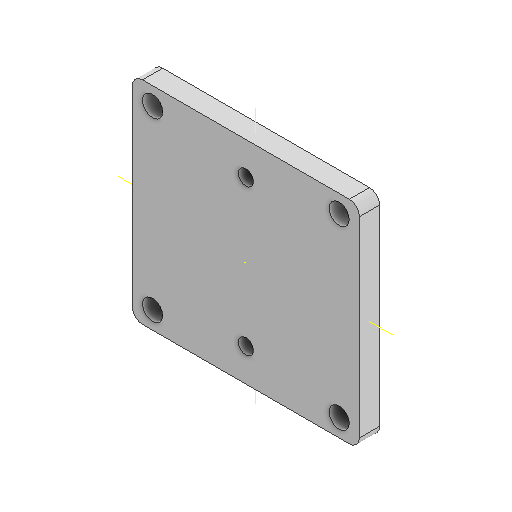
# Autodesk Inventor part: 집게_고정대
Saved by Autodesk Inventor 2027 (Build 310192000, 192)
## iProperties
Created: 2026-09-23
Part Number: 집게_고정대
Material: 일반
Document SubType Name: Modeling
Designer: User
Density: 1 g/cm^3
Appearance: 기본값
Author: User
Autodesk Inventor part; units mm, degrees
ref_plane "YZ 평면_우측면도" through (0, 0, 0) normal (1, 0, 0) x (0, 1, 0)
ref_plane "XZ 평면_평면도" through (0, 0, 0) normal (0, 1, 0) x (-1, 0, 0)
ref_plane "XY 평면_정면도" through (0, 0, 0) normal (0, 0, 1) x (1, 0, 0)
sketch "스케치1" plane through (0, 0, 0) normal (0, 0, 1) x (1, 0, 0)
  line L0 (20.5, -21) -> (-20.5, -21)
  line L1 (-22.5, -19) -> (-22.5, 19)
  line L2 (-20.5, 21) -> (20.5, 21)
  line L3 (22.5, 19) -> (22.5, -19)
  line L4 (22.5, -21) -> (-22.5, 21) construction
  line L5 (-22.5, -21) -> (22.5, 21) construction
  line L6 (0, 21) -> (0, -21) construction
  line L7 (-22.5, 14.5) -> (22.5, 14.5) construction
  circle A0 centre (0, 14.5) radius 1.5
  line L8 (-22.5, -14.5) -> (22.5, -14.5) construction
  circle A1 centre (0, -14.5) radius 1.5
  line L9 (-23.5, -17.5) -> (26.5, -17.5) construction
  line L10 (-23.5, 17.5) -> (26.5, 17.5) construction
  line L11 (-18.5, 21) -> (-18.5, -21) construction
  line L12 (18.5, 21) -> (18.5, -21) construction
  circle A2 centre (-18.5, 17.5) radius 2
  circle A3 centre (-18.5, -17.5) radius 2
  circle A4 centre (18.5, 17.5) radius 2
  circle A5 centre (18.5, -17.5) radius 2
  line L13 (-33.5, 0) -> (36.5, 0) projected
  line L14 (0, -29.9799) -> (0, 29.9799) projected
  arc A6 (-20.5, 21) -> (-22.5, 19) centre (-20.5, 19) ccw
  arc A7 (-22.5, -19) -> (-20.5, -21) centre (-20.5, -19) ccw
  arc A8 (20.5, -21) -> (22.5, -19) centre (20.5, -19) ccw
  arc A9 (22.5, 19) -> (20.5, 21) centre (20.5, 19) ccw
  point P0 (0, 0)
  dimension "d26" = 3
  dimension "d27" = 4
  dimension "d28" = 4
  dimension "d29" = 4
  dimension "d30" = 3
  dimension "d31" = 4
  dimension "d32" = 29
  dimension "d33" = 18.5
  dimension "d34" = 35
  dimension "d35" = 42
  dimension "d36" = 45
  dimension "d37" = 2
  constraints: 32 point on line, 26 end point, 10 centre point, 8 point on circle, 8 tangent, 6 midpoint, 4 parallel, 3 equal radius, 3 perpendicular, 2 horizontal, 1 collinear, 3 other
  measures "d26" diameter of A0
  measures "d27" diameter of A2
  measures "d28" diameter of A4
  measures "d29" diameter of A3
  measures "d30" diameter of A1
  measures "d31" diameter of A5
  measures "d32" distance between parallel lines of L8 L7
  measures "d33" distance between parallel lines of L6 L11
  measures "d34" distance between parallel lines of L9 L10
  measures "d35" distance between parallel lines of L0 L2
  measures "d36" distance between parallel lines of L3 L1
  measures "d37" radius of A6
extrude "돌출1" add sketch "스케치1" along normal mid plane 4 contours L0 L14 A1 L13 L3 A8 | L0 A7 L1 L13 L14 A1 | L13 L14 A0 L2 A9 L3 | L13 L1 A6 L2 L14 A0
